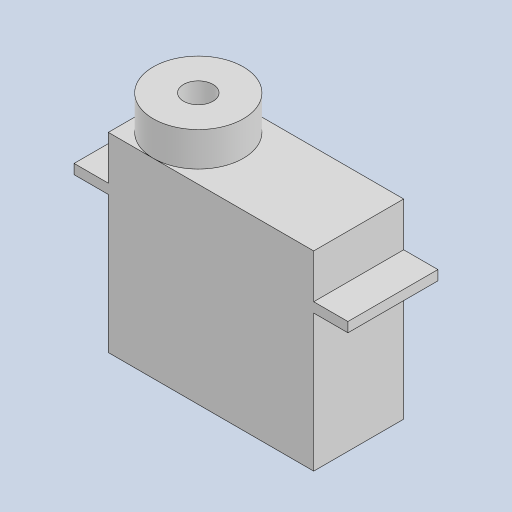
# Autodesk Inventor part: motor
Saved by Autodesk Inventor 2023 (Build 270158000, 158)
## iProperties
Created: 2022-06-06
Part Number: motor
Material: Generic
Document SubType Name: Modeling
Designer: legot
Density: 1 g/cm^3
Appearance: Default
Author: legot
Autodesk Inventor part; units mm, degrees
ref_plane "YZ Plane" through (0, 0, 0) normal (1, 0, 0) x (0, 1, 0)
ref_plane "XZ Plane" through (0, 0, 0) normal (0, 1, 0) x (-1, 0, 0)
ref_plane "XY Plane" through (0, 0, 0) normal (0, 0, 1) x (1, 0, 0)
sketch "スケッチ1" plane through (0, 0, 0) normal (0, 1, 0) x (-1, 0, 0)
  line L0 (0, 0) -> (-21, 0)
  line L1 (-21, 0) -> (-21, -9.2)
  line L2 (-21, -9.2) -> (0, -9.2)
  line L3 (0, -9.2) -> (0, 0)
  dimension "d0" = 21
  dimension "d1" = 9.2
  constraints: 8 end point, 2 parallel, 1 horizontal, 1 perpendicular
  measures "d0" distance of L1.end L2.end
  measures "d1" distance of L0.end L1.end
extrude "押し出し1" add sketch "スケッチ1" along normal blind 14
sketch "スケッチ2" plane through (0, 14, 0) normal (0, 1, 0) x (1, 0, 0)
  line L0 (21, 0) -> (21, 9.2) projected
  line L1 (21, 9.2) -> (0, 9.2) projected
  line L2 (0, 9.2) -> (0, 0) projected
  line L3 (0, 0) -> (21, 0) projected
  line L4 (-3.5, 0) -> (24.5, 0)
  line L5 (24.5, 0) -> (24.5, 9.2)
  line L6 (24.5, 9.2) -> (-3.5, 9.2)
  line L7 (-3.5, 9.2) -> (-3.5, 0)
  dimension "d4" = 3.5
  dimension "d5" = 3.5
  constraints: 8 end point, 2 collinear, 2 parallel, 1 horizontal, 1 perpendicular
  measures "d4" distance between parallel lines of L7 L2
  measures "d5" distance between parallel lines of L0 L5
extrude "押し出し2" add sketch "スケッチ2" along normal blind 1
sketch "スケッチ3" plane through (0, 15, 0) normal (0, 1, 0) x (1, 0, 0)
  line L0 (-3.5, 0) -> (24.5, 0) projected
  line L1 (24.5, 9.2) -> (-3.5, 9.2) projected
  line L2 (0, 9.2) -> (0, 0) projected
  line L3 (21, 0) -> (21, 9.2) projected
extrude "押し出し3" add sketch "スケッチ3" along normal blind 4.5
sketch "スケッチ4" plane through (0, 19.5, 0) normal (0, 1, 0) x (1, 0, 0)
  line L0 (21, 9.2) -> (0, 9.2) projected
  line L1 (0, 9.2) -> (0, 0) projected
  line L2 (0, 0) -> (21, 0) projected
  circle A0 centre (4.6, 4.6) radius 4.6
  constraints: 3 tangent, 1 centre point
extrude "押し出し4" add sketch "スケッチ4" along normal blind 3.5 contours A0
sketch "スケッチ5" plane through (4.6, 23, -4.6) normal (0, 1, 0) x (1, 0, 0)
  circle A0 centre (0, 0) radius 4.6 projected
  point P0 (-4.6, -4.6)
  constraints: 1 coincident
hole "穴1" at (4.6, 23, -4.6) direction (0, -1, 0) diameter 3 end through all
equation "\"d5\" = d4"
